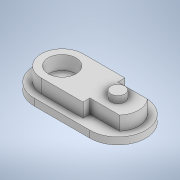
# Autodesk Inventor part: PivotLock
Saved by Autodesk Inventor 2022.2 (Build 262287030, 287C)
## iProperties
Created: 2023-04-24
Part Number: PivotLock
Material: Generic
Document SubType Name: Modeling
Designer: jak27277
Density: 1 g/cm^3
Appearance: Default
Mass: 59.0518 g
Surface Area: 150.657 cm^2
Volume: 59.0518 cm^3
Author: jak27277
Autodesk Inventor part; units mm, degrees
ref_plane "YZ Plane" through (0, 0, 0) normal (1, 0, 0) x (0, 1, 0)
ref_plane "XZ Plane" through (0, 0, 0) normal (0, 1, 0) x (-1, 0, 0)
ref_plane "XY Plane" through (0, 0, 0) normal (0, 0, 1) x (1, 0, 0)
sketch "Sketch1" plane through (0, 0, 0) normal (0, 1, 0) x (-1, 0, 0)
  line L0 (25.4, 0) -> (-25.4, 0) construction
  line L1 (25.4, 25.4) -> (-25.4, 25.4)
  line L2 (-25.4, -25.4) -> (25.4, -25.4)
  arc A0 (25.4, -25.4) -> (25.4, 25.4) centre (25.4, 0) ccw
  arc A1 (-25.4, 25.4) -> (-25.4, -25.4) centre (-25.4, 0) ccw
  point P0 (0, 0)
  dimension "d0" = 50.8
  dimension "d1" = 25.4
  constraints: 8 end point, 4 point on circle, 4 tangent, 2 centre point, 1 horizontal, 1 midpoint, 1 parallel
  measures "d0" distance of L2.start L2.end
  measures "d1" radius of A1
extrude "Extrusion1" add sketch "Sketch1" along normal blind 6.35
sketch "Sketch2" plane through (0, 6.35, 0) normal (0, 1, 0) x (1, 0, 0)
  line L0 (25.4, 0) -> (-25.4, 0) construction
  line L1 (25.4, 19.05) -> (-25.4, 19.05)
  line L2 (-25.4, -19.05) -> (25.4, -19.05)
  arc A0 (25.4, -19.05) -> (25.4, 19.05) centre (25.4, 0) ccw
  arc A1 (-25.4, 19.05) -> (-25.4, -19.05) centre (-25.4, 0) ccw
  line L3 (25.4, 25.4) -> (-25.4, 25.4) projected
  line L4 (12.7, -19.05) -> (12.7, -12.7)
  line L5 (12.7, -12.7) -> (39.599, -12.7)
  line L6 (12.7, 19.05) -> (12.7, 12.7)
  line L7 (12.7, 12.7) -> (39.599, 12.7)
  circle A2 centre (-25.4, 0) radius 12.7
  point P0 (0, 0)
  point P1 (0, 0)
  point P2 (12.7, -15.875)
  point P3 (39.599, 12.7)
  dimension "d4" = 19.05
  dimension "d5" = 38.1
  dimension "d6" = 25.4
  dimension "d7" = 25.4
  constraints: 16 end point, 5 point on circle, 4 tangent, 3 centre point, 3 symmetric about line, 2 coincident, 2 midpoint, 2 parallel, 1 horizontal, 1 perpendicular, 1 point on line, 1 vertical
  measures "d4" radius of A1
  measures "d5" horizontal distance of point (12.7, -15.875) L2.start
  measures "d6" distance between parallel lines of L5 L7
  measures "d7" diameter of A2
extrude "Extrusion2" add sketch "Sketch2" along normal blind 12.7 contours L6 L7 A0 L5 L4 L2 A1 L1
sketch "Sketch3" plane through (0, 19.05, 0) normal (0, 1, 0) x (1, 0, 0)
  arc A0 (25.4, -25.4) -> (25.4, 25.4) centre (25.4, 0) ccw projected
  circle A1 centre (25.4, 0) radius 6.35
  point P0 (0, 0)
  dimension "d10" = 12.7
  constraints: 1 centre point, 1 coincident
  measures "d10" diameter of A1
extrude "Extrusion3" add sketch "Sketch3" along normal blind 6.35
body "Solid1"
